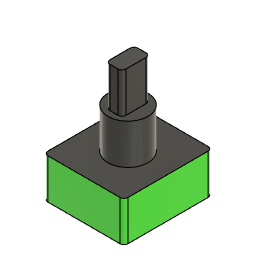
MG996R_Pot v2 (Autodesk Fusion 360 design; units mm, degrees)
Autodesk Fusion 360 part; units mm, degrees
sketch "Sketch1" plane through (0, 0, 0) normal (0, 0, 1) x (1, 0, 0)
  line L0 (5, 5.5) -> (-5, 5.5)
  line L1 (-5, 5.5) -> (-5, -5.5)
  line L2 (-5, -5.5) -> (5, -5.5)
  line L3 (5, -5.5) -> (5, 5.5)
  line L4 (5, 5.5) -> (-5, -5.5) construction
  line L5 (-5, 5.5) -> (5, -5.5) construction
  dimension "d1" = 10
  dimension "d2" = 11
  constraint horizontal L0
  constraint perpendicular L0 L1
  constraint parallel L0 L2
  constraint parallel L1 L3
  constraint coincident L4 origin
  constraint coincident L5 origin
  measures "d1" distance of L0.start L0.end
  measures "d2" distance of L0.end L1.end
extrude "Extrude1" add sketch "Sketch1" along normal blind 5
sketch "Sketch2" plane through (0, 0, 5) normal (0, 0, 1) x (-1, 0, 0)
  line L0 (-5, 5.5) -> (-5, -5.5)
  line L1 (-5, -5.5) -> (5, -5.5)
  line L2 (5, -5.5) -> (5, 5.5)
  line L3 (5, 5.5) -> (-5, 5.5)
  circle A0 centre (0, 0) radius 2.5
  dimension "d5" = 5
  constraint coincident A0.centre origin
  measures "d5" diameter of A0
extrude "Extrude2" add sketch "Sketch2" along normal blind 10 contours A0
sketch "Sketch3" plane through (0, 0, 15) normal (0, 0, 1) x (-1, 0, 0)
  circle A0 centre (0, 0) radius 2.5
  line L0 (-1, -1.75) -> (1, -1.75)
  line L1 (1, -1.75) -> (1, 1.75)
  line L2 (1, 1.75) -> (-1, 1.75)
  line L3 (-1, 1.75) -> (-1, -1.75)
  line L4 (-1, -1.75) -> (1, 1.75) construction
  line L5 (1, -1.75) -> (-1, 1.75) construction
  dimension "d8" = 2
  dimension "d9" = 3.5
  constraint horizontal L0
  constraint perpendicular L0 L1
  constraint parallel L0 L2
  constraint parallel L1 L3
  constraint coincident L4 A0.centre
  constraint coincident L5 A0.centre
  constraint coincident A0.centre origin
  measures "d8" distance of L1 L3
  measures "d9" distance of L0.end L1.end
extrude "Extrude3" cut sketch "Sketch3" against normal blind 5
fillet "Fillet1" radius 0.5 4 edges at (-1, -1.75, 12.5) (1, -1.75, 12.5) (-1, 1.75, 12.5) (1, 1.75, 12.5)
fillet "Fillet2" radius 0.5 4 edges at (-5, 5.5, 2.5) (5, 5.5, 2.5) (-5, -5.5, 2.5) (5, -5.5, 2.5)
